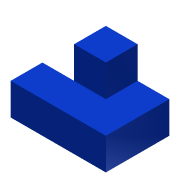
# Autodesk Inventor part: BluePuzzlePiece
Saved by Autodesk Inventor 2015 (Build 190159000, 159)
## iProperties
Created: 2016-10-14
Part Number: BluePuzzlePiece
Material: Generic
Document SubType Name: Modeling
Designer: Aniket Pant
Density: 1 g/cm^3
Appearance: Default
Mass: 98.3224 g
Surface Area: 154.838 cm^2
Volume: 98.3224 cm^3
Author: Aniket Pant
Autodesk Inventor part; units mm, degrees
ref_plane "YZ Plane" through (0, 0, 0) normal (1, 0, 0) x (0, 1, 0)
ref_plane "XZ Plane" through (0, 0, 0) normal (0, 1, 0) x (-1, 0, 0)
ref_plane "XY Plane" through (0, 0, 0) normal (0, 0, 1) x (1, 0, 0)
sketch "Sketch1" plane through (0, 0, 0) normal (0, 1, 0) x (-1, 0, 0)
  line L0 (0, 0) -> (76.2, 0)
  line L1 (76.2, 0) -> (76.2, -25.4)
  line L2 (76.2, -25.4) -> (50.8, -25.4)
  line L3 (50.8, -25.4) -> (50.8, -50.8)
  line L4 (50.8, -50.8) -> (0, -50.8)
  line L5 (0, -50.8) -> (0, 0)
  dimension "d0" = 76.2
  dimension "d1" = 25.4
  dimension "d2" = 25.4
  dimension "d3" = 25.4
  dimension "d4" = 50.8
  constraints: 12 end point, 4 perpendicular, 1 horizontal
  measures "d0" distance of L0.start L0.end
  measures "d1" distance of L0.end L1.end
  measures "d2" distance of L1.end L2.end
  measures "d3" distance of L2.end L3.end
  measures "d4" distance of L3.end L4.end
extrude "Extrusion1" add sketch "Sketch1" along normal blind 25.4
sketch "Sketch2" plane through (0, 25.4, 0) normal (0, 1, 0) x (1, 0, 0)
  line L0 (-50.8, 25.4) -> (-25.4, 25.4)
  line L1 (-25.4, 25.4) -> (-25.4, 50.8)
  line L2 (-25.4, 50.8) -> (-50.8, 50.8)
  line L3 (-50.8, 50.8) -> (-50.8, 25.4)
  line L4 (-50.8, 50.8) -> (-50.8, 25.4) projected
  point P0 (0, 0)
  dimension "d7" = 25.4
  constraints: 8 end point, 2 perpendicular, 1 collinear, 1 horizontal
  measures "d7" distance of L0.start L0.end
extrude "Extrusion2" add sketch "Sketch2" along normal blind 25.4
body "Solid1"
